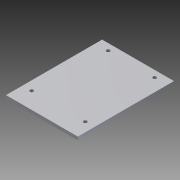
# Autodesk Inventor part: 20
Saved by Autodesk Inventor 2013 (Build 170138000, 138)
## iProperties
Created: 2013-12-19
Material: アセタール樹脂、白
Document SubType Name: シート メタル
Designer: andou
Density: 1.425 g/cm^3
Sheet Metal Rule: Default
Mass: 24.0376 g
Surface Area: 122.783 cm^2
Volume: 16.8685 cm^3
Part Number: 20
Author: andou
Title: Beagle_Bone_Plate
Autodesk Inventor part; units mm, degrees
ref_plane "YZ Plane" through (0, 0, 0) normal (1, 0, 0) x (0, 1, 0)
ref_plane "XZ Plane" through (0, 0, 0) normal (0, 1, 0) x (-1, 0, 0)
ref_plane "XY Plane" through (0, 0, 0) normal (0, 0, 1) x (1, 0, 0)
sketch "スケッチ1" plane through (0, 0, 0) normal (0, 0, 1) x (1, 0, 0)
  line L0 (-32.5, 43.5) -> (32.5, 43.5)
  line L1 (32.5, 43.5) -> (32.5, -43.5)
  line L2 (32.5, -43.5) -> (-32.5, -43.5)
  line L3 (-32.5, -43.5) -> (-32.5, 43.5)
  point P0 (0, 0)
  dimension "d0" = 87
  dimension "d1" = 65
  dimension "d2" = 32.5
  dimension "d3" = 43.5
  constraints: 8 end point, 2 parallel, 1 horizontal, 1 perpendicular
  measures "d0" distance of L2.end L0.start
  measures "d1" distance of L1.end L2.end
  measures "d2" distance from line of point (0, 0) L3
  measures "d3" distance from line of L2 point (0, 0)
extrude "押し出し1" add sketch "スケッチ1" along normal blind 3
sketch "スケッチ2" plane through (0, 0, 3) normal (0, 0, 1) x (1, 0, 0)
  circle A0 centre (-21, 37.5) radius 1.6
  circle A1 centre (21, 37.5) radius 1.6
  circle A2 centre (-24.25, -28.5) radius 1.6
  circle A3 centre (24.25, -28.5) radius 1.6
  point P0 (0, 0)
  dimension "d6" = 3.2
  dimension "d7" = 42
  dimension "d8" = 48.5
  dimension "d9" = 24.25
  dimension "d10" = 21
  dimension "d11" = 66
  dimension "d12" = 66
  dimension "d52" = 28.5
  dimension "d53" = 28.5
  constraints: 4 centre point, 3 equal radius
  measures "d6" diameter of A1
  measures "d7" distance of A1.centre A0.centre
  measures "d8" distance of A3.centre A2.centre
  measures "d9" horizontal distance of point (0, 0) A2.centre
  measures "d10" horizontal distance of A1.centre point (0, 0)
  measures "d11" vertical distance of A3.centre A1.centre
  measures "d12" vertical distance of A0.centre A2.centre
  measures "d52" vertical distance of point (0, 0) A2.centre
  measures "d53" vertical distance of A3.centre point (0, 0)
hole "穴1" at (-24.25, -28.5, 3) at (24.25, -28.5, 3) at (21, 37.5, 3) at (-21, 37.5, 3) direction (0, 0, -1) diameter 3.2 end through all
equation "\"BendRadius\" = 厚さ"
equation "\"BendReliefWidth\" = 厚さ"
equation "\"BendReliefDepth\" = 0.5 * 厚さ"
equation "\"CornerReliefSize\" = 4 * 厚さ"
equation "\"MinimumRemnant\" = 2 * 厚さ"
equation "\"TransitionRadius\" = BendRadius"
equation "\"JacobiRadiusSize\" = 厚さ"
equation "\"GapSize\" = 厚さ"
equation "\"厚さ\" = 0.5"
